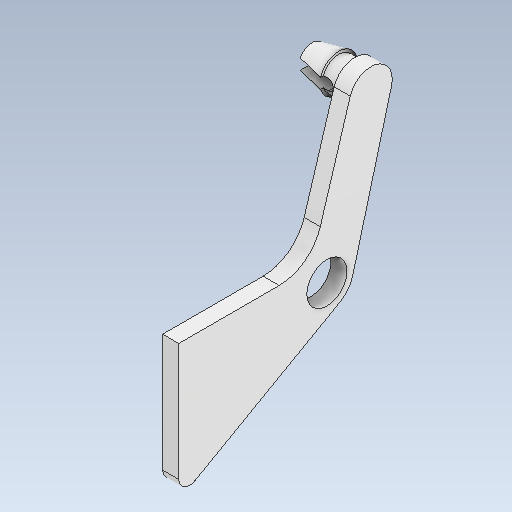
# Autodesk Inventor part: trigger
Saved by Autodesk Inventor 2021 (Build 250183000, 183)
## iProperties
Created: 2023-08-11
Part Number: trigger
Material: Plástico PPS
Document SubType Name: Modeling
Designer: Sergio
Density: 1.637 g/cm^3
Appearance: Suave - Blanco
Author: Sergio
Autodesk Inventor part; units mm, degrees
ref_plane "YZ Plane" through (0, 0, 0) normal (1, 0, 0) x (0, 1, 0)
ref_plane "XZ Plane" through (0, 0, 0) normal (0, 1, 0) x (-1, 0, 0)
sketch "Boceto4" plane through (0, 0, 0) normal (1, 0, 0) x (0, 1, 0)
  line L0 (0, 0) -> (0, 25.2)
  line L1 (0, 0) -> (26.7765, -8.1864)
  line L2 (0, 0) -> (28, 0) construction
  line L3 (4, 25.2) -> (4, 2.9598)
  line L4 (4, 2.9598) -> (27.946, -4.3612)
  circle A0 centre (26.7765, -8.1864) radius 4
  circle A1 centre (0, 0) radius 4.976
  line L5 (0, 25.2) -> (-20, 25.2)
  line L6 (-20, 25.2) -> (-4.3292, -2.4533)
  line L7 (25.7411, -12.0501) -> (-1.2881, -4.8064)
  line L8 (4, 25.2) -> (4, 27.6)
  line L9 (4, 27.6) -> (-17.9279, 27.6)
  line L10 (-19.6679, 24.6139) -> (-20, 25.2)
  arc A2 (-17.9279, 27.6) -> (-19.6679, 24.6139) centre (-17.9279, 25.6) ccw
  circle A3 centre (0, 0) radius 3.75
  point P0 (-19.8875, 25.2)
  point P1 (-19.6679, 24.6139)
  dimension "d18" = 25.2
  dimension "d20" = 28
  dimension "d22" = 4
  dimension "d23" = 20
  dimension "d24" = 2.4
  dimension "d25" = 2
  dimension "d26" = 7.5
  dimension "d44" = 107
  dimension "d45" = 2.4
  constraints: 22 end point, 7 point on circle, 6 tangent, 4 centre point, 3 coincident, 2 horizontal, 2 vertical, 1 collinear, 1 equal length, 1 perpendicular, 1 other
  measures "d18" distance of L0.start L0.end
  measures "d20" distance of L0.start L1.end
  measures "d22" distance between parallel lines of L0 L3
  measures "d23" distance of L0.end L5.end
  measures "d24" distance of L3.start L8.end
  measures "d25" radius of A2
  measures "d26" diameter of A3
  measures "d44" angle of L0 L1
  measures "d45" distance between parallel lines of L5 L9
extrude "Extrusión2" add sketch "Boceto4" along normal mid plane 3 contours A3 L1 A1 L0 | L0 A1 L1 A3 | A1 L6 A2 L5 L0 | L0 L5 A2 L9 L8 L3 A1 | A1 L4 A0 L1 | L1 A0 L7 A1 | A0
fillet "Empalme1" radius 8 1 edges at (0, 4, 2.9598)
ref_plane "Plano de trabajo3" through (0, 0, -8.1864) normal (0, 0, 1) x (1, 0, 0)
sketch "Boceto5" plane through (0, 0, -8.1864) normal (0, 0, 1) x (1, 0, 0)
  line L0 (0, 0) -> (0, 26.7765)
  line L1 (0, 26.7765) -> (-1.5, 26.7765)
  line L2 (-1.5, 26.7765) -> (-1.5, 23.7765)
  line L3 (-1.5, 30.7765) -> (-1.5, 25.7411) projected
  line L4 (-1.5, 23.7765) -> (-4.5, 23.7765)
  line L5 (-4.5, 23.7765) -> (-4.5, 23.2765)
  line L6 (-4.5, 23.2765) -> (-9.5, 23.2765)
  line L7 (-9.5, 23.2765) -> (-9.5, 26.7765)
  line L8 (-9.5, 26.7765) -> (-9.5, 24.4033)
  line L9 (-9.5, 24.4033) -> (-4.5, 23.2765)
  line L10 (-9.5, 26.7765) -> (-1.5, 26.7765)
  point P0 (-1.5, 27.946)
  dimension "d31" = 26.7765
  dimension "d32" = 1.5
  dimension "d33" = 3
  dimension "d34" = 3
  dimension "d35" = 0.5
  dimension "d36" = 5
  dimension "d37" = 3.5
  dimension "d38" = 2.3732
  constraints: 20 end point, 2 horizontal, 2 perpendicular, 2 vertical, 1 collinear, 1 point on line
  measures "d31" distance of L0.start L0.end
  measures "d32" distance of L0.end L1.end
  measures "d33" distance of L1.end L2.end
  measures "d34" distance of L2.end L4.end
  measures "d35" distance of L4.end L5.end
  measures "d36" distance of L5.end L6.end
  measures "d37" distance of L6.end L7.end
  measures "d38" distance of L7.end L8.end
revolve "Revolución1" add sketch "Boceto5" angle 360 about axis through (-9.5, 26.7765, -8.1864) along (1, 0, 0) contours L2 L4 L5 L9 L7 L10
ref_plane "Plano de trabajo4" through (-3, 26.7765, -11.1864) normal (0, 0, 1) x (1, 0, 0)
sketch "Boceto6" plane through (-3, 26.7765, -11.1864) normal (0, 0, 1) x (1, 0, 0)
  line L0 (-6.5, 2.3732) -> (-6.5, -2.3732) projected
  line L1 (-6.5, 0) -> (-3, 0)
  line L2 (0.5, 1) -> (-6.5, 1)
  line L3 (-6.5, 1) -> (-6.5, -1)
  line L4 (-6.5, -1) -> (0.5, -1)
  line L5 (0.5, -1) -> (0.5, 1)
  line L6 (0.5, 1) -> (-6.5, -1) construction
  line L7 (-6.5, 1) -> (0.5, -1) construction
  point P0 (3, -26.7765)
  point P1 (-6.5, 1)
  dimension "d40" = 3.5
  dimension "d41" = 2
  constraints: 14 end point, 3 midpoint, 2 horizontal, 2 parallel, 1 perpendicular, 1 point on line
  measures "d40" distance of L1.start L1.end
  measures "d41" distance of L3.end L2.end
extrude "Extrusión3" cut sketch "Boceto6" against normal mid plane 14
fillet "Empalme2" radius 1 2 edges at (-2.5, 27.7765, -8.1864) (-2.5, 25.7765, -8.1864)
equation "\"d45\" = d24"
equation "\"offset\" = 1"
equation "\"thikness\" = 2"
equation "\"r1\" = 5.55"
equation "\"r2o\" = 59.75"
equation "\"delta_y\" = 6"
equation "\"wire_d\" = 1"
equation "\"width_ang_spring\" = 5"
equation "\"spring_int_diam\" = 8.5"
equation "\"spring_ext_diam\" = 10.5"
equation "\"r3\" = 8.25"
equation "\"r3R\" = 4.75"
equation "\"r3T\" = 6.74537"
equation "\"alpha\" = 54.847297deg"
equation "\"alpha2\" = 270deg"
equation "\"theta3_recogido\" = 305.152703deg"
equation "\"delta_theta_3\" = 45deg"
equation "\"joint_width\" = 12"
equation "\"joint_radius\" = 7.75"
equation "\"shaft_width\" = 15"
equation "\"shaft_joint_diameter\" = 7.75"
equation "\"separation_space\" = 0.5"
equation "\"height_finger\" = 42"
equation "\"cell_screw_head_diameter\" = 4"
equation "\"cell_screw_diameter\" = 2"
equation "\"cell_space\" = 2"
equation "\"cell_width\" = 6"
equation "\"cell_theta_position\" = 60deg"
equation "\"cell_thikness\" = 1"
equation "\"cell_lenght\" = 37"
equation "\"cell_z_space\" = 5"
equation "\"wire_D\" = 2.3"
equation "\"width_link\" = 8"
equation "\"Dt\" = 1.05949"
equation "\"Djoint_shaft\" = 2.3"
equation "\"shaft_x\" = 1.45"
equation "\"shaft_y\" = 6.45"
equation "\"lenght_body_link\" = 186.05"
equation "\"lenght_bar_support\" = 201.65"
equation "\"wire_spring_d\" = 1"
equation "\"spring_int_d\" = 6"
equation "\"spring_lenght\" = 28"
equation "\"trigger_offset\" = 2"
equation "\"e\" = 9"
equation "\"So\" = 17"
equation "\"m2_theta3o\" = -30deg"
equation "\"m2_r3\" = 19.75"
equation "\"m2_delta_theta1\" = 15deg"
equation "\"m2_theta3f\" = -60deg"
equation "\"trigger_thumb_lenght\" = 6"
equation "\"r3_thikness\" = 3.5"
equation "\"tg_width\" = 4"
equation "\"pivot_screw_d\" = 4"
equation "\"sf_lenght\" = 9.5"
equation "\"sf_base\" = 3"
equation "\"sf_head_height\" = 3"
equation "\"sf_head_width\" = 4.5"
equation "\"sf_head_offset\" = 0.25"
equation "\"sf_head_grip_width\" = 2"
equation "\"sf_head_angle\" = 45deg"
equation "\"sf_thikness\" = 5"
equation "\"screw_Dhead\" = 8"
equation "\"screw_d\" = 4"
equation "\"screw_lenght\" = 12"
equation "\"screwJ_base_D\" = 9"
equation "\"screwJ_top_D\" = 13"
equation "\"gj_D\" = 6"
equation "\"gj_d\" = 4"
equation "\"gj_out_section\" = 6"
equation "\"ext_width_slider\" = 3.5"
equation "\"sfbox_tip_width\" = 2.5"
equation "\"slim_width_slider\" = 1.5"
equation "\"agarradera_width\" = 4"
equation "\"int_width_slider\" = 2"
equation "\"agarradera_position\" = 82.13077"
equation "\"sfbox_theta1\" = 60deg"
equation "\"sfbox_theta2\" = 45deg"
equation "\"agarradera_theta\" = 60deg"
equation "\"sfbox_width\" = 1.5"
equation "\"box_fat_slider_lenght\" = 67"
equation "\"fat_width_slider\" = 2"
equation "\"box_in_width\" = 72"
equation "\"flex_separation_theta\" = 60deg"
equation "\"sf_flex_separation\" = 38.66667"
equation "\"thikness_box\" = 1.5"
equation "\"box_slim_slider_lenght\" = 116"
equation "\"box_in_deep\" = 77"
equation "\"box_in_height\" = 35"
